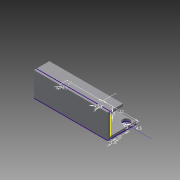
# Autodesk Inventor part: TopClip
Saved by Autodesk Inventor 2014 SP1 (Build 180222100, 222)
## iProperties
Created: 2015-03-31
Part Number: TopClip
Material: Generic
Document SubType Name: Modeling
Designer: Erin
Density: 1 g/cm^3
Appearance: Default
Author: Erin
Autodesk Inventor part; units mm, degrees
ref_plane "YZ Plane" through (0, 0, 0) normal (1, 0, 0) x (0, 1, 0)
ref_plane "XZ Plane" through (0, 0, 0) normal (0, 1, 0) x (-1, 0, 0)
ref_plane "XY Plane" through (0, 0, 0) normal (0, 0, 1) x (1, 0, 0)
sketch "Sketch1" plane through (0, 0, 0) normal (0, 0, 1) x (1, 0, 0)
  circle A0 centre (0, 0) radius 2.25
  circle A1 centre (-19.75, 0) radius 2.25
  circle A2 centre (19.75, 0) radius 2.25
  line L0 (0, 13.6364) -> (0, -14.2241) construction
  line L1 (-36.2718, 0) -> (35.3009, 0) construction
  line L2 (-22.75, 3) -> (22.75, 3)
  line L3 (22.75, 3) -> (22.75, -3)
  line L4 (22.75, -3) -> (-22.75, -3)
  line L5 (-22.75, -3) -> (-22.75, 3)
  line L6 (-22.75, -3) -> (22.75, -3)
  line L7 (22.75, -3) -> (22.75, -13)
  line L8 (22.75, -13) -> (-22.75, -13)
  line L9 (-22.75, -13) -> (-22.75, -3)
  line L10 (-22.75, -13) -> (22.75, -13)
  line L11 (22.75, -13) -> (22.75, -14.5)
  line L12 (22.75, -14.5) -> (-22.75, -14.5)
  line L13 (-22.75, -14.5) -> (-22.75, -13)
  dimension "d0" = 4.5
  dimension "d1" = 4.5
  dimension "d2" = 4.5
  dimension "d5" = 3
  dimension "d6" = 3
  dimension "d7" = 3
  dimension "d8" = 3
  dimension "d9" = 10
  dimension "d10" = 1.5
  dimension "d20" = 22
  dimension "d21" = 22
  constraints: 28 end point, 6 parallel, 4 horizontal, 4 perpendicular, 3 centre point, 2 collinear, 2 point on line, 2 vertical, 1 coincident
  measures "d0" diameter of A0
  measures "d1" diameter of A1
  measures "d2" diameter of A2
  measures "d5" distance from line of A0.centre L2
  measures "d6" distance from line of A0.centre L4
  measures "d7" distance from line of A2.centre L3
  measures "d8" distance from line of A1.centre L5
  measures "d9" distance of L6.end L7.end
  measures "d10" distance of L10.end L11.end
extrude "Extrusion1" add sketch "Sketch1" along normal blind 1.5
extrude "Extrusion2" add sketch "Sketch1" along normal blind 13.5 contours L8 L11 L12 L13
sketch "Sketch2" plane through (-22.75, -13, 1.5) normal (0, 1, 0) x (1, 0, 0)
  line L0 (45.5, 0) -> (45.5, -12) projected
  line L1 (0, -12) -> (45.5, -12)
  line L2 (45.5, -12) -> (45.5, -13.5)
  line L3 (45.5, -13.5) -> (0, -13.5)
  line L4 (0, -13.5) -> (0, -12)
  point P0 (22.75, 1.5)
  dimension "d15" = 1.5
  constraints: 8 end point, 2 parallel, 1 collinear, 1 horizontal, 1 perpendicular
  measures "d15" distance of L1.end L2.end
extrude "Extrusion3" add sketch "Sketch2" against normal blind 1.5
extrude "Extrusion4" add sketch "Sketch2" along normal blind 8
body "Solid1"
